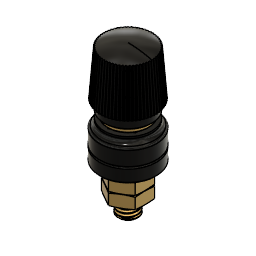
M6 100A Binding Post Black v3 (Autodesk Fusion 360 design; units mm, degrees)
Autodesk Fusion 360 part; units mm, degrees
sketch "Sketch1" plane through (0, 0, 0) normal (0, 1, 0) x (1, 0, 0)
  circle A0 centre (0, 0) radius 3
  dimension "d1" = 6
  constraint coincident A0.centre origin
  measures "d1" diameter of A0
extrude "Extrude1" add sketch "Sketch1" against normal blind 17.4 makes body 1
extrude "Extrude2" add 1 faces at (-1.1591, 0, -0.5829) along direction (0, 1, 0) blind 15 on bodies 1 bodies 1
chamfer "Chamfer1" distance 0.4 angle 45 2 edges at (-2.797, -17.4, -1.0848) (-2.797, 15, 1.0848) on bodies 1
thread "Thread1" "ISO Metric profile 6.0 M6x1 M6x1 6g" major diameter 5.884 minor diameter 4.7435 pitch 1 angle 60 modelled right hand crest width 0.1444 on face at (2.9851, -6.4667, 0.2987) crest through (2.942, 14.85, 0) on bodies 1
sketch "Sketch2" plane through (0, 0, 0) normal (0, 0, 1) x (1, 0, 0)
  line L0 (-3.1, 0) -> (-3.1, 7)
  line L1 (-3.1, 7) -> (-7, 7)
  line L2 (-7, 7) -> (-7, 5)
  line L3 (-7, 5) -> (-8.3, 5)
  line L4 (-8.3, 5) -> (-8.3, 0)
  line L5 (-8.3, 0) -> (-3.1, 0)
  line L6 (0, 0) -> (0, 7) construction
  line L7 (-3.1, 7) -> (0, 7) construction
  dimension "d9" = 7
  dimension "d10" = 3.1
  dimension "d11" = 8.3
  dimension "d13" = 7
  dimension "d22" = 2
  constraint vertical L0
  constraint perpendicular L0 L1
  constraint perpendicular L1 L2
  constraint perpendicular L2 L3
  constraint perpendicular L3 L4
  constraint perpendicular L0 L5
  constraint coincident L6.start origin
  constraint perpendicular L1 L6
  constraint perpendicular L6 L7
  measures "d9" distance of L0.start L0.end
  measures "d10" distance of L6.start L0.start
  measures "d11" distance of L6.start L4.end
  measures "d13" distance of L1.end L6.end
  measures "d22" distance of L1 L3
revolve "Revolve1" add sketch "Sketch2" angle 360 about axis through (0, 0, 0) along (0, 1, 0) separate body makes body 2
sketch "Sketch3" plane through (0, 7, 0) normal (0, 1, 0) x (-1, 0, 0)
  circle A0 centre (0, 0) radius 7
  circle A1 centre (0, 0) radius 3.1
  line L0 (5.05, 2.9156) -> (0, 5.8312)
  line L1 (0, 5.8312) -> (-5.05, 2.9156)
  line L2 (-5.05, 2.9156) -> (-5.05, -2.9156)
  line L3 (-5.05, -2.9156) -> (0, -5.8312)
  line L4 (0, -5.8312) -> (5.05, -2.9156)
  line L5 (5.05, -2.9156) -> (5.05, 2.9156)
  line L6 (0, 0) -> (0, 5.8312) construction
  dimension "d15" = 10.1
  constraint coincident A0.centre A1.centre
  constraint vertical L6
  measures "d15" distance of L2 L5
extrude "Extrude3" cut sketch "Sketch3" against normal blind 3.5 contours L0 L1 L2 L3 L4 L5 bodies 2
fillet "Fillet1" radius 1.5 1 edges at (-6.5263, 5, 2.5313) on bodies 2
fillet "Fillet2" radius 0.8 1 edges at (-7.7383, 5, 3.0014) on bodies 2
sketch "Sketch4" plane through (0, 0, 0) normal (0, -1, 0) x (1, 0, 0)
  circle A0 centre (0, 0) radius 3.1
  circle A1 centre (0, 0) radius 8.3
  circle A2 centre (0, 0) radius 4.5
  dimension "d24" = 9
  constraint coincident A0.centre A1.centre
  measures "d24" diameter of A2
extrude "Extrude4" cut sketch "Sketch4" against normal blind 2 contours A2 bodies 2
fillet "Fillet4" radius 0.3 11 edges at (-7.7383, 0, 3.0014) (-4.1955, 0, 1.6273) (-4.1955, 2, 1.6273) (2.8902, 2, 1.121) (2.8902, 3.5, -1.121) (2.525, 3.5, -4.3734) (-2.525, 3.5, -4.3734) (5.05, 3.5, 0) (2.525, 3.5, 4.3734) (-2.525, 3.5, 4.3734) (-5.05, 3.5, 0) on bodies 2
sketch "Sketch5" plane through (0, 0, 0) normal (0, 1, 0) x (1, 0, 0)
  line L0 (4.95, 2.8579) -> (0, 5.7158)
  line L1 (0, 5.7158) -> (-4.95, 2.8579)
  line L2 (-4.95, 2.8579) -> (-4.95, -2.8579)
  line L3 (-4.95, -2.8579) -> (0, -5.7158)
  line L4 (0, -5.7158) -> (4.95, -2.8579)
  line L5 (4.95, -2.8579) -> (4.95, 2.8579)
  line L6 (0, 0) -> (0, 5.7158) construction
  circle A0 centre (0, 0) radius 3
  dimension "d27" = 9.9
  dimension "d28" = 6
  constraint coincident L6.start A0.centre
  constraint vertical L6
  measures "d27" distance of L2 L5
  measures "d28" diameter of A0
extrude "Extrude5" add sketch "Sketch5" along normal blind 3.6 separate body makes body 3
sketch "Sketch6" plane through (0, 0, 0) normal (0, 0, 1) x (1, 0, 0)
  line L0 (-3, 3.6) -> (3, 3.6)
  line L1 (4.95, 3.6) -> (0, 3.6)
  line L2 (0, 3.6) -> (-4.95, 3.6)
  line L3 (-4.95, 3.6) -> (0, 3.6)
  line L4 (0, 3.6) -> (4.95, 3.6)
  line L5 (6.8, 3.6) -> (6.8, 3.1)
  line L6 (4.8, 3.6) -> (6.8, 3.1)
  line L7 (4.8, 3.6) -> (3.9569, 3.8108)
  line L8 (3.9569, 3.8108) -> (6.7992, 3.8108)
  line L9 (6.7992, 3.8108) -> (6.8, 3.6)
  dimension "d31" = 0.5
  dimension "d32" = 6.8
  dimension "d33" = 2
  constraint coincident L4 L6.start
  constraint parallel L4 L8
  constraint collinear L6 L7
  measures "d31" distance of L5.start L5.end
  measures "d32" distance of L1.end L5
  measures "d33" distance of L5 L6.start
revolve "Revolve2" cut sketch "Sketch6" angle 360 about axis through (0, 1.75, 0) along (0, 1, 0) contours L5 L6 L7 L8 L9 in plane through (0, 0, 0.001) normal (0, 0.000284, 1) bodies 3
ref_plane "WorkPlane1" through (0, 1.8, 0.0055) normal (0, 1, 0) x (1, 0, 0)
mirror "Mirror1" about plane through (0, 1.8, 0.0055) normal (0, 1, 0) of "Revolve2"
thread "Thread2" "ISO Metric profile 6.0 M6x1 M6x1 6H" major diameter 6.147 minor diameter 5.035 pitch 1 angle 60 modelled right hand crest width 0.2748 on face at (2.9851, 1.2, 0.2987) crest through (2.5175, 0.25, 0) on bodies 3
copy_body "Body->Comp1" bodies 3 removing the originals makes body 4 in component "M6 Thin Nut"
sketch "Sketch7" plane through (0, 0, 0) normal (0, 1, 0) x (1, 0, 0)
  circle A0 centre (0, 0) radius 8.3
  circle A1 centre (0, 0) radius 3.1
  circle A2 centre (0, 0) radius 4.3
  dimension "d43" = 16.6
  dimension "d44" = 6.2
  dimension "d45" = 8.6
  constraint coincident A0.centre A1.centre
  constraint concentric A0 A1
  measures "d43" diameter of A0
  measures "d44" diameter of A1
  measures "d45" diameter of A2
extrude "Extrude6" add sketch "Sketch7" against normal blind 4 separate body contours A0 | A2 makes body 5
extrude "Extrude7" add sketch "Sketch7" along normal blind 2 contours A2 bodies 5
fillet "Fillet3" radius 0.3 3 edges at (-7.7383, -4, -3.0014) (-7.7383, 0, 3.0014) (-4.009, 0, -1.5549) 1 faces at (3.8724, 2, 0.3676) on bodies 5
sketch "Sketch8" plane through (0, -4, 0) normal (0, -1, 0) x (1, 0, 0)
  circle A0 centre (0, 0) radius 3.1
  circle A1 centre (0, 0) radius 8
  circle A2 centre (0, 0) radius 6
  circle A3 centre (0, 0) radius 3.15
  dimension "d54" = 12
  dimension "d55" = 6.3
  constraint coincident A0.centre A1.centre
  constraint concentric A2 A3
  measures "d54" diameter of A2
  measures "d55" diameter of A3
extrude "Extrude8" add sketch "Sketch8" along normal blind 1.6 separate body contours A2 makes body 6
fillet "Fillet5" radius 0.3 1 faces at (5.0277, -5.6, -0.2981) on bodies 6
copy_body "Body->Comp2" bodies 6 removing the originals makes body 7 in component "M6 Washer"
copy_body "Body->Comp3" bodies 5 removing the originals makes body 8 in component "Inner Base"
copy_body "Body->Comp4" bodies 1 removing the originals makes body 9 in component "M6 Bar"
copy_body "Body->Comp5" bodies 2 removing the originals makes body 10 in component "Outer Base"
sketch "Sketch9" plane through (0, 0, 0) normal (0, 0, 1) x (1, 0, 0)
  line L0 (0, 0) -> (8.15, 0) construction
  line L1 (8.15, 0) -> (8.15, 17.3) construction
  line L2 (0, 16.2) -> (8.15, 16.2) construction
  line L3 (7, 0) -> (7, 3)
  line L4 (7, 3) -> (8.15, 3)
  line L5 (3, 0) -> (3, 10)
  line L6 (3, 10) -> (0, 10)
  line L7 (8.15, 3) -> (7.15, 16.2)
  line L8 (0, 10) -> (0, 17.2)
  line L9 (3, 0) -> (7, 0)
  spline S0 degree 5 poles (0, 17.2) (0.1765, 17.2) (0.53, 17.1965) (1.0615, 17.1807) (1.7706, 17.1397) (2.6441, 17.0603) (3.4868, 16.9596) (4.2797, 16.8442) (5.006, 16.7202) (5.6566, 16.5919) (6.2315, 16.4617) (6.6333, 16.3571) (6.9035, 16.2786) (7.0701, 16.2262) (7.15, 16.2) knots 0 0 0 0 0 0 0.1 0.2 0.3 0.4 0.5 0.6 0.7 0.8 0.9 1 1 1 1 1 1
  line L10 (-0.7708, 17.2) -> (0.7708, 17.2)
  point P0 (4.7008, 16.77)
  dimension "d88" = 17.2
  dimension "d90" = 1
  dimension "d91" = 10
  dimension "d93" = 3
  dimension "d95" = 1
  dimension "d113" = 8.15
  dimension "d114" = 7
  constraint coincident L0.start origin
  constraint perpendicular L0 L1
  constraint coincident L1 L2.end
  constraint perpendicular L1 L2
  constraint coincident L0 L3.start
  constraint perpendicular L0 L3
  constraint coincident L1 L4.end
  constraint perpendicular L1 L4
  constraint coincident L0 L5.start
  constraint perpendicular L0 L5
  constraint coincident L2 L7.end
  constraint midpoint L8.end L10
  constraint horizontal L10
  constraint coincident L8.end S0.start
  measures "d88" distance of L0.start L8.end
  measures "d90" distance of L8.end L2
  measures "d91" distance of L5.start L5.end
  measures "d93" distance of L3.start L3.end
  measures "d95" distance of L2.end L7.end
  measures "d113" distance of L0.start L1
  measures "d114" distance of L0.start L3
revolve "Revolve3" add sketch "Sketch9" angle 360 about axis through (0, 10, 0) along (0, 1, 0) separate body makes body 11
sketch "Sketch10" plane through (0, 0, 0) normal (0, 0, 1) x (1, 0, 0)
  line L0 (6.9594, 18.7155) -> (8.4561, -1.0407)
  point P0 (8.15, 3)
  point P1 (7.15, 16.2)
  constraint coincident P1 L0
  constraint coincident P0 L0
ref_plane "WorkPlane2" through (6.9594, 18.7155, 0) normal (0.075541, -0.997143, 0) x (0.997143, 0.075541, 0)
sketch "Sketch11" plane through (6.9594, 18.7155, 0) normal (0.075541, -0.997143, 0) x (0.997143, 0.075541, 0)
  line L0 (0.3, -0.6) -> (0.3, 0.6)
  line L1 (0.3, 0.6) -> (-0.3, 0)
  line L2 (-0.3, 0) -> (0.3, -0.6)
  line L3 (0, 0) -> (0.3, 0) construction
  line L4 (-0.3, 0) -> (0, 0) construction
  dimension "d98" = 1.2
  dimension "d99" = 0.6
  dimension "d102" = 0.3
  constraint vertical L0
  constraint coincident L3.start L4.end
  constraint midpoint L0 L3.end
  constraint horizontal L3
  constraint horizontal L4
  measures "d98" distance of L0.start L0.end
  measures "d99" distance of L0 L1.end
  measures "d102" distance of L3.start L0
extrude "Extrude9" cut sketch "Sketch11" along normal blind 18 bodies 11
pattern_circular "C-Pattern1" count 60 over 360 about axis through (0, 1.75, 0) along (0, 1, 0) of "Extrude9"
thread "Thread3" "ISO Metric profile 6.0 M6x1 M6x1 6H" major diameter 6.147 minor diameter 5.035 pitch 1 angle 60 modelled right hand crest width 0.2748 on face at (2.9612, 3.3333, 0.4812) crest through (2.5175, 9.75, 0) on bodies 11
fillet "Fillet6" radius 0.3 2 edges at (-6.5263, 0, -2.5313) (-6.5263, 3, -2.5313) on bodies 11
copy_body "Body->Comp6" bodies 11 removing the originals makes body 12 in component "Cap"
component "M6 Thin Nut" placed x (1, 0, 0) y (0, 1, 0) z (0, 0, 1) at (0, 3.5, -0.0055)
component "M6 Washer" placed x (1, 0, 0) y (0, 1, 0) z (0, 0, 1) at (0, 0, 0)
component "Inner Base" placed x (1, 0, 0) y (0, 1, 0) z (0, 0, 1) at (0, 0, 0)
component "M6 Bar" placed x (1, 0, 0) y (0, 1, 0) z (0, 0, 1) at (0, 0, 0)
component "Outer Base" placed x (1, 0, 0) y (0, 1, 0) z (0, 0, 1) at (0, 0, 0)
component "M6 Washer" placed x (1, 0, 0) y (0, 1, 0) z (0, 0, 1) at (0, 12.7, 0)
component "M6 Thin Nut" placed x (1, 0, 0) y (0, 1, 0) z (0, 0, 1) at (0, -12.8, -0.0055)
component "M6 Thin Nut" placed x (1, 0, 0) y (0, 1, 0) z (0, 0, 1) at (0, -9.2, -0.0055)
component "Cap" placed x (1, 0, 0) y (0, 1, 0) z (0, 0, 1) at (0, 8.7, 0)
named bodies: "M6 Bar", "Outer Base", "M6 Thin Nut", "Inner Base", "M6 Washer", "Cap"
